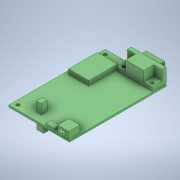
# Autodesk Inventor part: Spo2 PCB
Saved by Autodesk Inventor 2020 (Build 240168000, 168)
## iProperties
Created: 2021-04-18
Part Number: Spo2 PCB
Material: Generic
Document SubType Name: Modeling
Designer: Karl
Density: 1 g/cm^3
Appearance: Smooth - Dark Forest Green
Author: Karl
Autodesk Inventor part; units mm, degrees
ref_plane "YZ Plane" through (0, 0, 0) normal (1, 0, 0) x (0, 1, 0)
ref_plane "XZ Plane" through (0, 0, 0) normal (0, 1, 0) x (-1, 0, 0)
ref_plane "XY Plane" through (0, 0, 0) normal (0, 0, 1) x (1, 0, 0)
sketch "Sketch1" plane through (0, 0, 0) normal (0, 1, 0) x (-1, 0, 0)
  line L0 (-26.9875, 42.8625) -> (26.9875, 42.8625)
  line L1 (26.9875, 42.8625) -> (26.9875, -42.8625)
  line L2 (26.9875, -42.8625) -> (-26.9875, -42.8625)
  line L3 (-26.9875, -42.8625) -> (-26.9875, 42.8625)
  line L4 (-26.9875, 42.8625) -> (26.9875, -42.8625) construction
  line L5 (26.9875, 42.8625) -> (-26.9875, -42.8625) construction
  point P0 (0, 0)
  dimension "d0" = 53.975
  dimension "d1" = 85.725
  constraints: 12 end point, 2 midpoint, 2 parallel, 1 horizontal, 1 perpendicular
  measures "d0" distance of L1.end L2.end
  measures "d1" distance of L0.end L1.end
extrude "Extrusion1" add sketch "Sketch1" along normal blind 1.57
sketch "Sketch2" plane through (0, 1.57, 0) normal (0, 1, 0) x (1, 0, 0)
  line L0 (-26.9875, -42.8625) -> (26.9875, -42.8625) projected
  line L1 (-26.9875, 42.8625) -> (-26.9875, -42.8625) projected
  line L2 (26.9875, 42.8625) -> (-26.9875, 42.8625) projected
  line L3 (26.9875, -42.8625) -> (26.9875, 42.8625) projected
  point P0 (0, 0)
  point P1 (-22.9235, -38.7985)
  point P2 (-22.9235, 38.7985)
  dimension "d4" = 4.064
  dimension "d5" = 4.064
  dimension "d6" = 4.064
  dimension "d7" = 4.064
  measures "d4" distance from line of L0 point (-22.923, -38.798)
  measures "d5" distance from line of L1 point (-22.923, -38.798)
  measures "d6" distance from line of L1 point (-22.923, 38.798)
  measures "d7" distance from line of point (-22.923, 38.798) L2
hole "Hole1" at (-22.9235, 1.57, 38.7985) at (-22.9235, 1.57, -38.7985) direction (0, -1, 0) diameter 3 depth 2.54
sketch "Sketch5" plane through (0, 1.57, 0) normal (0, 1, 0) x (1, 0, 0)
  line L0 (-26.9875, -42.8625) -> (26.9875, -42.8625) projected
  line L1 (26.9875, -42.8625) -> (26.9875, 42.8625) projected
  line L2 (-4.9284, -30.8693) -> (-9.1184, -30.8693)
  line L3 (-9.1184, -30.8693) -> (-9.1184, -36.0693)
  line L4 (-9.1184, -36.0693) -> (-4.9284, -36.0693)
  line L5 (-4.9284, -36.0693) -> (-4.9284, -30.8693)
  line L6 (-4.9284, -30.8693) -> (-9.1184, -36.0693) construction
  line L7 (-9.1184, -30.8693) -> (-4.9284, -36.0693) construction
  point P0 (0, 0)
  point P1 (-7.3025, -33.9725)
  point P2 (-7.0234, -33.4693)
  dimension "d26" = 8.89
  dimension "d27" = 34.29
  dimension "d28" = 5.2
  dimension "d29" = 4.19
  constraints: 12 end point, 2 midpoint, 2 parallel, 1 horizontal, 1 perpendicular
  measures "d26" distance from line of point (-7.303, -33.973) L0
  measures "d27" distance from line of L1 point (-7.303, -33.973)
  measures "d28" distance of L2.end L3.end
  measures "d29" distance of L3.end L4.end
extrude "Extrusion4" add sketch "Sketch5" along normal blind 8.77
sketch "Sketch6" plane through (0, 1.57, 0) normal (0, 1, 0) x (1, 0, 0)
  line L0 (-6.0004, 7.1846) -> (-24.0004, 7.1846)
  line L1 (-24.0004, 7.1846) -> (-24.0004, 32.6846)
  line L2 (-24.0004, 32.6846) -> (-6.0004, 32.6846)
  line L3 (-6.0004, 32.6846) -> (-6.0004, 7.1846)
  line L4 (-6.0004, 7.1846) -> (-24.0004, 32.6846) construction
  line L5 (-24.0004, 7.1846) -> (-6.0004, 32.6846) construction
  point P0 (0, 0)
  point P1 (-15.0004, 19.9346)
  dimension "d34" = 25.5
  dimension "d35" = 18
  constraints: 12 end point, 2 midpoint, 2 parallel, 1 horizontal, 1 perpendicular
  measures "d34" distance of L0.end L1.end
  measures "d35" distance of L0.start L0.end
extrude "Extrusion5" add sketch "Sketch6" along normal blind 4.2
sketch "Sketch7" plane through (0, 0, 0) normal (0, -1, 0) x (1, 0, 0)
  line L0 (2.7595, 37.1835) -> (-3.1405, 37.1835)
  line L1 (-3.1405, 37.1835) -> (-3.1405, 41.6835)
  line L2 (-3.1405, 41.6835) -> (2.7595, 41.6835)
  line L3 (2.7595, 41.6835) -> (2.7595, 37.1835)
  line L4 (2.7595, 37.1835) -> (-3.1405, 41.6835) construction
  line L5 (-3.1405, 37.1835) -> (2.7595, 41.6835) construction
  line L6 (-26.9875, 42.8625) -> (26.9875, 42.8625) projected
  line L7 (-26.9875, -42.8625) -> (-26.9875, 42.8625) projected
  line L8 (26.9875, 42.8625) -> (26.9875, -42.8625) projected
  point P0 (0, 0)
  point P1 (-0.1905, 39.4335)
  dimension "d36" = 4.5
  dimension "d37" = 5.9
  dimension "d38" = 3.429
  dimension "d40" = 27.178
  constraints: 12 end point, 2 midpoint, 2 parallel, 1 horizontal, 1 perpendicular
  measures "d36" distance of L2.end L0.start
  measures "d37" distance of L0.start L0.end
  measures "d38" distance from line of L6 point (-0.191, 39.433)
  measures "d40" distance from line of L8 point (-0.191, 39.433)
extrude "Extrusion6" add sketch "Sketch7" along normal blind 6
sketch "Sketch8" plane through (0, 1.57, 0) normal (0, 1, 0) x (1, 0, 0)
  line L0 (26.0985, -42.6085) -> (16.2941, -42.6085)
  line L1 (16.2941, -42.6085) -> (16.2941, -32.7279)
  line L2 (16.2941, -32.7279) -> (26.0985, -32.7279)
  line L3 (26.0985, -32.7279) -> (26.0985, -42.6085)
  line L4 (26.0985, -42.6085) -> (16.2941, -32.7279) construction
  line L5 (16.2941, -42.6085) -> (26.0985, -32.7279) construction
  line L6 (26.9875, -42.8625) -> (26.9875, 42.8625) projected
  line L7 (-26.9875, -42.8625) -> (26.9875, -42.8625) projected
  point P0 (0, 0)
  point P1 (21.1963, -37.6682)
  dimension "d43" = 9.8044
  dimension "d44" = 9.8806
  dimension "d45" = 0.889
  dimension "d46" = 0.254
  constraints: 12 end point, 2 midpoint, 2 parallel, 1 horizontal, 1 perpendicular
  measures "d43" distance of L1.end L2.end
  measures "d44" distance of L0.end L1.end
  measures "d45" distance between parallel lines of L6 L3
  measures "d46" distance between parallel lines of L0 L7
extrude "Extrusion7" add sketch "Sketch8" along normal blind 6.1722
sketch "Sketch9" plane through (16.2941, 1.57, 42.6085) normal (0, 0, 1) x (1, 0, 0)
  line L0 (0, 0) -> (0, 6.1722) projected
  line L1 (7.0358, 4.2799) -> (2.2606, 4.2799)
  line L2 (2.2606, 4.2799) -> (2.2606, 1.8923)
  line L3 (2.2606, 1.8923) -> (7.0358, 1.8923)
  line L4 (7.0358, 1.8923) -> (7.0358, 4.2799)
  line L5 (7.0358, 4.2799) -> (2.2606, 1.8923) construction
  line L6 (2.2606, 4.2799) -> (7.0358, 1.8923) construction
  line L7 (0, 6.1722) -> (9.8044, 6.1722) projected
  point P0 (-16.2941, -1.57)
  point P1 (4.6482, 3.0861)
  dimension "d52" = 3.0861
  dimension "d53" = 2.2606
  constraints: 12 end point, 2 midpoint, 2 parallel, 1 horizontal, 1 perpendicular
  measures "d52" distance from line of L7 point (4.648, 3.086)
  measures "d53" distance between parallel lines of L0 L2
extrude "Extrusion8" add sketch "Sketch9" along normal blind 2.4892
sketch "Sketch10" plane through (0, 1.57, 0) normal (0, 1, 0) x (1, 0, 0)
  line L0 (26.9875, -42.8625) -> (26.9875, 42.8625) projected
  line L1 (-26.9875, -42.8625) -> (26.9875, -42.8625) projected
  line L2 (13.0175, -42.2275) -> (5.3975, -42.2275)
  line L3 (5.3975, -42.2275) -> (5.3975, -37.1475)
  line L4 (5.3975, -37.1475) -> (13.0175, -37.1475)
  line L5 (13.0175, -37.1475) -> (13.0175, -42.2275)
  line L6 (13.0175, -42.2275) -> (5.3975, -37.1475) construction
  line L7 (5.3975, -42.2275) -> (13.0175, -37.1475) construction
  point P0 (0, 0)
  point P1 (9.2075, -39.6875)
  dimension "d56" = 17.78
  dimension "d57" = 3.175
  dimension "d58" = 7.62
  dimension "d59" = 5.08
  constraints: 12 end point, 2 midpoint, 2 parallel, 1 horizontal, 1 perpendicular
  measures "d56" distance from line of L0 point (9.208, -39.688)
  measures "d57" distance from line of L1 point (9.208, -39.688)
  measures "d58" distance of L3.end L4.end
  measures "d59" distance of L2.end L3.end
extrude "Extrusion9" add sketch "Sketch10" along normal blind 1.8
sketch "Sketch11" plane through (0, 1.57, 0) normal (0, 1, 0) x (1, 0, 0)
  line L0 (26.9875, -42.8625) -> (26.9875, 42.8625) projected
  line L1 (26.9875, 42.8625) -> (-26.9875, 42.8625) projected
  circle A0 centre (23.3172, 34.1249) radius 1.524
  circle A1 centre (-1.6764, 34.1249) radius 1.524
  point P0 (0, 0)
  dimension "d62" = 3.6703
  dimension "d63" = 24.9936
  dimension "d64" = 8.7376
  dimension "d65" = 8.7376
  dimension "d66" = 3.048
  dimension "d67" = 3.048
  constraints: 2 centre point, 2 coincident
  measures "d62" distance from line of point (23.317, 34.125) L0
  measures "d63" distance of point (-1.676, 34.125) point (23.317, 34.125)
  measures "d64" distance from line of L1 point (23.317, 34.125)
  measures "d65" distance from line of L1 point (-1.676, 34.125)
  measures "d66" diameter of A0
  measures "d67" diameter of A1
sketch "Sketch12" plane through (0, 1.57, 0) normal (0, 1, 0) x (1, 0, 0)
  line L0 (26.9875, -42.8625) -> (26.9875, 42.8625) projected
  line L1 (26.9875, 34.1249) -> (26.2255, 34.1249)
  line L2 (26.9875, 34.1249) -> (27.7495, 34.1249) construction
  line L3 (26.9875, 42.8625) -> (-26.9875, 42.8625) projected
  line L4 (26.2255, 34.1249) -> (26.2255, 31.1785)
  line L5 (26.2255, 31.1785) -> (-4.5847, 31.1785)
  line L6 (-4.5847, 31.1785) -> (-4.5847, 43.6245)
  line L7 (-4.5847, 43.6245) -> (26.2255, 43.6245)
  line L8 (26.2255, 43.6245) -> (26.2255, 31.1785)
  point P0 (0, 0)
  point P1 (26.2255, 42.8625)
  point P2 (-4.5847, 42.8625)
  dimension "d68" = 0.762
  dimension "d69" = 180
  dimension "d70" = 8.7376
  dimension "d73" = 2.9464
  dimension "d74" = 30.8102
  dimension "d75" = 12.446
  constraints: 14 end point, 2 horizontal, 2 parallel, 2 perpendicular, 1 collinear, 1 point on line
  measures "d68" distance of L1.start L1.end
  measures "d69" angle of L1 L2
  measures "d70" distance between parallel lines of L3 L1
  measures "d73" distance of L1.end L4.end
  measures "d74" distance of L6.end L7.end
  measures "d75" distance of L5.end L6.end
extrude "Extrusion10" add sketch "Sketch12" along normal blind 12.5476 contours L4 L5 L6 L3 L8 | L3 L6 L7 L8
sketch "Sketch15" plane through (26.2255, 1.57, -43.6245) normal (0, 0, -1) x (-1, 0, 0)
  line L0 (23.5585, 2.3241) -> (7.2517, 2.3241)
  line L1 (7.2517, 2.3241) -> (7.2517, 10.2235)
  line L2 (7.2517, 10.2235) -> (23.5585, 10.2235)
  line L3 (23.5585, 10.2235) -> (23.5585, 2.3241)
  line L4 (23.5585, 2.3241) -> (7.2517, 10.2235) construction
  line L5 (7.2517, 2.3241) -> (23.5585, 10.2235) construction
  line L6 (30.8102, 0) -> (30.8102, 12.5476) projected
  line L7 (0, 12.5476) -> (30.8102, 12.5476) projected
  point P0 (26.2255, -1.57)
  point P1 (26.9875, 0)
  point P2 (15.4051, 6.2738)
  point P3 (30.8102, 6.2738)
  point P4 (15.4051, 12.5476)
  dimension "d86" = 16.3068
  dimension "d87" = 7.8994
  constraints: 12 end point, 4 midpoint, 2 parallel, 1 horizontal, 1 perpendicular
  measures "d86" distance of L1.end L2.end
  measures "d87" distance of L0.end L1.end
extrude "Extrusion13" add sketch "Sketch15" along normal blind 6.0452
sketch "Sketch16" plane through (0, 14.1176, 0) normal (0, 1, 0) x (1, 0, 0)
  line L0 (26.2255, 43.6245) -> (-4.5847, 43.6245) projected
  line L1 (-1.9136, 43.6245) -> (-1.9136, 40.0431)
  line L2 (-1.9136, 43.6245) -> (1.6678, 43.6245) construction
  line L3 (22.654, 43.6245) -> (22.654, 40.0431)
  line L4 (26.2255, 42.8625) -> (26.2255, 31.1785) projected
  line L5 (18.9738, 43.6245) -> (18.9738, 49.6697) projected
  line L6 (26.2255, 31.1785) -> (-4.5847, 31.1785) projected
  line L7 (-4.5847, 43.6245) -> (-4.5847, 31.1785) projected
  line L8 (2.667, 43.6245) -> (2.667, 49.6697) projected
  line L9 (18.9738, 40.0431) -> (26.2255, 40.0431)
  line L10 (18.9738, 40.0431) -> (18.9738, 31.1785)
  line L11 (2.667, 40.0431) -> (-4.5847, 40.0431)
  line L12 (-4.5847, 31.1785) -> (-4.5847, 42.8625) projected
  line L13 (2.667, 40.0431) -> (2.667, 31.1785)
  point P0 (0, 0)
  dimension "d90" = 3.5814
  dimension "d91" = 270
  dimension "d92" = 3.5814
  constraints: 14 end point, 8 point on line, 6 perpendicular, 1 horizontal
  measures "d90" distance of L1.start L1.end
  measures "d92" distance of L3.start L3.end
extrude "Extrusion14" cut sketch "Sketch16" against normal blind 8.9662 contours L9 L4 L6 L10 | L11 L13 L6 L7
extrude "Extrusion15" cut sketch "Sketch11" along normal mid plane 8.9662
body "Solid1"
